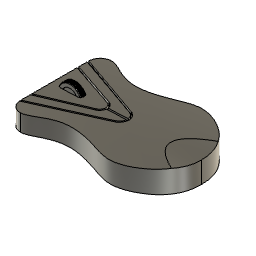
A4_AI22BTECH11005_4 (Autodesk Fusion 360 design; units mm, degrees)
Autodesk Fusion 360 part; units mm, degrees
sketch "Sketch1" plane through (0, 0, 0) normal (0, 0, 1) x (1, 0, 0)
  line L0 (0, 30) -> (0, -30)
  arc A0 (0, -30) -> (10, -40) centre (10, -30) ccw
  arc A1 (10, 40) -> (0, 30) centre (10, 30) ccw
  spline S0 degree 5 poles (10, 40) (10.9946, 40) (13.0682, 39.7459) (16.4315, 38.6027) (21.4876, 35.8702) (29.0437, 32.0592) (38.0149, 29.581) (48.2736, 29.5355) (59.1098, 31.6881) (69.5734, 35.0916) (78.8703, 38.4218) (86.7641, 40.4007) (93.9362, 40.1363) (102.6229, 37.6436) (112.4243, 32.71) (121.8387, 25.096) (127.3679, 16.6467) (129.5519, 8.8878) (130.0159, 3.0701) (130, 0) knots 0 0 0 0 0 0 0.066667 0.133333 0.2 0.266667 0.333333 0.4 0.466667 0.533333 0.6 0.666667 0.733333 0.8 0.866667 0.933333 1 1 1 1 1 1
  line L1 (2.9289, 40) -> (17.0711, 40)
  line L2 (27.8536, 31.0429) -> (52.1464, 28.9571)
  line L3 (82.1526, 40.1526) -> (97.8474, 39.8474)
  line L4 (130, 0) -> (0, 0)
  spline S1 degree 5 poles (10, -40) (10.9946, -40) (13.0682, -39.7459) (16.4315, -38.6027) (21.4876, -35.8702) (29.0437, -32.0592) (38.0149, -29.581) (48.2736, -29.5355) (59.1098, -31.6881) (69.5734, -35.0916) (78.8703, -38.4218) (86.7641, -40.4007) (93.9362, -40.1363) (102.6229, -37.6436) (112.4243, -32.71) (121.8387, -25.096) (127.3679, -16.6467) (129.5519, -8.8878) (130.0159, -3.0701) (130, 0) knots 0 0 0 0 0 0 0.066667 0.133333 0.2 0.266667 0.333333 0.4 0.466667 0.533333 0.6 0.666667 0.733333 0.8 0.866667 0.933333 1 1 1 1 1 1
  line L5 (130.0753, 14.5031) -> (129.9247, -14.5031)
  line L6 (2.9289, -40) -> (17.0711, -40)
  line L7 (27.8536, -31.0429) -> (52.1464, -28.9571)
  line L8 (82.1526, -40.1526) -> (97.8474, -39.8474)
  line L9 (130.0753, -14.5031) -> (129.9247, 14.5031)
  arc A2 (0, -30) -> (10, -40) centre (10, -30) ccw
  line L10 (0, -30) -> (0, 30)
  point P0 (130, 0)
  point P1 (40, 30)
  point P2 (90, 40)
  point P3 (40, -30)
  point P4 (90, -40)
  dimension "d1" = 10
  constraint vertical L0
  constraint tangent L0 A0
  constraint tangent L0 A1
  constraint equal A0 A1
  constraint coincident P0 S0.end
  constraint midpoint A1.start L1
  constraint tangent A1 L1
  constraint midpoint P1 L2
  constraint midpoint P2 L3
  constraint coincident L4.end origin
  constraint perpendicular L0 L4
  constraint midpoint P0 L5
  constraint symmetric L0.end L4 L0.start
  constraint symmetric L0.start L4 L0.end
  constraint symmetric A1.start L4 A0.end
  constraint symmetric A1 L4 A2
  constraint symmetric P1 L4 P3
  constraint symmetric P2 L4 P4
  constraint symmetric L1.start L4 L6.start
  constraint symmetric L1.end L4 L6.end
  constraint symmetric L2.start L4 L7.start
  constraint symmetric L2.end L4 L7.end
  constraint symmetric L3.start L4 L8.start
  constraint symmetric L3.end L4 L8.end
  constraint symmetric L4 L5.start L9.start
  constraint symmetric L4 L5.end L9.end
  measures "d1" radius of A0
extrude "Extrude1" add sketch "Sketch1" against normal blind 20
sketch "Sketch2" plane through (0, 0, 0) normal (0, 1, 0) x (1, 0, 0)
  line L0 (0, 0) -> (130.3347, 0)
  line L1 (130.3347, 0) -> (130.3347, 5.593)
  line L2 (130.3347, 5.593) -> (0, 5.593)
  line L3 (0, 5.593) -> (0, 0)
  line L4 (0, 5.593) -> (0, 0)
  line L5 (130.3347, 0) -> (130.3347, 5.593)
  line L6 (130.3347, 0) -> (65.1673, 0)
  line L7 (0, 5.593) -> (130.3347, 0)
  constraint coincident L0.start L3.end
  constraint horizontal L0
  constraint perpendicular L0 L1
  constraint perpendicular L1 L2
  constraint perpendicular L0 L3
  constraint midpoint L0 L6.end
extrude "Extrude2" cut sketch "Sketch2" along normal mid plane 100 contours L0 L3 L4 L6 L7
sketch "Sketch3" plane through (0, 0, 0) normal (0, 0, 1) x (1, 0, 0)
  line L0 (-1.0692, 29.9861, -8.2811) -> (-1.1456, -30.0143, -8.2905)
  line L1 (-1.0692, 29.9861, -8.2811) -> (61.0097, 7.0411, -0.6588)
  line L2 (61.0097, -7.0411, -0.6588) -> (-1.1456, -30.0143, -8.2905)
  arc A0 through (61.0097, -7.0411, -0.6588) (65.8899, 0, -0.0596) (61.0097, 7.0411, -0.6588)
  line L3 (0, -20) -> (0, 20)
  line L4 (0, -20) -> (42.0778, -4.699)
  line L5 (42.0778, 4.699) -> (0, 20)
  arc A1 (42.0778, -4.699) -> (42.0778, 4.699) centre (40.3691, 0) ccw
  line L6 (-1.3, -21.856) -> (-1.3, 21.856)
  line L7 (42.5221, 5.9207) -> (-1.3, 21.856)
  arc A2 (42.5221, -5.9207) -> (42.5221, 5.9207) centre (40.3691, 0) ccw
  line L8 (-1.3, -21.856) -> (42.5221, -5.9207)
  line L9 (46.6691, 0, 0) -> (65.8899, 0, -0.0596)
  line L10 (65.8024, 0) -> (65.8024, -0.75)
  line L11 (65.8024, -0.75) -> (45.9997, -0.75)
  line L12 (65.8024, 0.75) -> (65.8024, 0)
  line L13 (45.9997, 0.75) -> (45.9997, -0.75)
  line L14 (45.9997, 0.75) -> (65.8024, 0.75)
  line L15 (8.5721, 2.853) -> (23.7087, 2.853)
  line L16 (26.2087, 0.353) -> (26.2087, -0.647)
  line L17 (23.7087, -3.147) -> (8.5721, -3.147)
  line L18 (6.0721, 0.353) -> (6.0721, -0.647)
  arc A3 (8.5721, 2.853) -> (6.0721, 0.353) centre (8.5721, 0.353) ccw
  arc A4 (26.2087, 0.353) -> (23.7087, 2.853) centre (23.7087, 0.353) ccw
  arc A5 (23.7087, -3.147) -> (26.2087, -0.647) centre (23.7087, -0.647) ccw
  arc A6 (6.0721, -0.647) -> (8.5721, -3.147) centre (8.5721, -0.647) ccw
  line L19 (6.0721, -0.0328) -> (26.2087, -0.0328)
  line L20 (16.1404, -0.0328) -> (16.1404, 2.4672)
  line L21 (16.1404, -0.0328) -> (16.1404, -2.5328)
  line L22 (65.8024, 0, 0) -> (-0.9655, -29.9477, -8.2684)
  line L23 (85, 0, 0) -> (-1.1453, -29.7384, -8.2905)
  point P0 (66.9185, 0)
  point P1 (45.0032, -0.0207)
  point P2 (26.2087, 2.853)
  point P3 (26.2087, -3.147)
  point P4 (108.295, 0)
  dimension "d6" = 7.5
  dimension "d10" = 40
  dimension "d11" = 5
  dimension "d12" = 1.3
  dimension "d14" = 0.75
  dimension "d18" = 6
  dimension "d22" = 2.5
  dimension "d23" = 2.5
  dimension "d24" = 2.5
  constraint vertical L3
  constraint tangent L4 A1
  constraint tangent L5 A1
  constraint perpendicular L11 L13
  constraint horizontal L15
  constraint perpendicular L15 L16
  constraint perpendicular L16 L17
  constraint perpendicular L17 L18
  constraint tangent L15 A3
  constraint tangent L18 A3
  constraint coincident P2 L15
  constraint coincident P2 L16
  constraint tangent L15 A4
  constraint tangent L16 A4
  constraint equal A3 A4
  constraint coincident P3 L16
  constraint coincident P3 L17
  constraint tangent L16 A5
  constraint tangent L17 A5
  constraint equal A3 A5
  constraint tangent L17 A6
  constraint tangent L18 A6
  constraint equal A3 A6
  constraint coincident L18 L19.start
  constraint coincident L16 L19.end
  constraint perpendicular L16 L19
  constraint midpoint L19 L20.start
  constraint perpendicular L15 L20
  constraint perpendicular L19 L21
  measures "d10" distance of L3.start L3.end
  measures "d11" radius of A1
  measures "d14" distance of L10.start L10.end
  measures "d18" distance of P2 P3
  measures "d22" radius of A3
  measures "d23" distance of L20.start L20.end
  measures "d24" distance of L20.start L21.end
extrude "Extrude4" cut sketch "Sketch3" along normal mid plane 14 contours L6 L7 A2 L8 L11 L13 L14 | A2 L11 L13 L14 | A2 L10 L11 L12 L14
extrude "Extrude5" cut sketch "Sketch3" against normal blind 12 contours L15 L16 L18 A3 A4 L19 | L16 L17 L18 A5 A6 L19
ref_plane "WorkPlane1" through (16.1404, 1.2172, 0) normal (1, 0, 0) x (0, 1, 0)
sketch "Sketch5" plane through (16.1404, 1.2172, 0) normal (1, 0, 0) x (0, 1, 0)
  line L0 (1.25, 0) -> (1.25, -1.9482)
  line L1 (1.25, 0) -> (1.25, 1)
  line L2 (-3.75, 0) -> (-3.75, 1)
  line L3 (-3.75, 0) -> (-3.75, -1.9758)
  line L4 (-2.75, -9) -> (0.25, -9)
  arc A0 (1.25, 1) -> (0.75, 1.5) centre (0.75, 1) ccw
  arc A1 (-3.25, 1.5) -> (-3.75, 1) centre (-3.25, 1) ccw
  line L5 (1.25, -1.9482) -> (0.25, -1.9482)
  line L6 (0.25, -1.9482) -> (0.25, -9)
  line L7 (-3.75, -1.9758) -> (-2.75, -1.9758)
  line L8 (-2.75, -1.9758) -> (-2.75, -9)
  line L9 (-1.93, -1.5) -> (-2.0076, -1.5)
  line L10 (-2.9954, -1.4863) -> (-2.9954, 1.5)
  line L11 (-2.4997, -1.4863) -> (-2.4997, 1.5)
  line L12 (0.5056, 1.5) -> (0.5056, -1.4863)
  line L13 (0.017, 1.5) -> (0.017, -1.4863)
  line L14 (-0.5066, 1.5) -> (-0.5066, -1.4863)
  line L15 (-1.0186, 1.5) -> (-1.0186, -1.4863)
  line L16 (-1.5189, 1.5) -> (-1.5189, -1.4863)
  line L17 (-2.0076, 1.5) -> (-2.0076, -1.5)
  line L18 (0.75, 1.5) -> (0.5056, 1.5)
  line L19 (0.017, 1.5) -> (-0.5066, 1.5)
  line L20 (-1.0186, 1.5) -> (-1.5189, 1.5)
  line L21 (-2.0076, 1.5) -> (-2.4997, 1.5)
  line L22 (-2.9954, 1.5) -> (-3.25, 1.5)
  line L23 (0.017, -1.4863) -> (0.5056, -1.4863)
  line L24 (-1.0186, -1.4863) -> (-0.5066, -1.4863)
  line L25 (-2.9954, -1.4863) -> (-2.4997, -1.4863)
  line L26 (-2.0076, -1.4863) -> (-1.5189, -1.4863)
  point P0 (-3.75, 0)
  point P1 (1.25, 0)
  point P2 (1.25, 1.5)
  point P3 (-3.75, 1.5)
  dimension "d47" = 1.5
  dimension "d48" = 0.5
  dimension "d49" = 0.5
  dimension "d65" = 1
  dimension "d66" = 1
  constraint coincident P1 L0.start
  constraint vertical L0
  constraint parallel L0 L1
  constraint coincident P0 L2.start
  constraint vertical L2
  constraint parallel L2 L3
  constraint perpendicular L0 L4
  constraint coincident P2 L1
  constraint tangent L1 A0
  constraint coincident P3 L2
  constraint tangent L2 A1
  constraint perpendicular L0 L5
  constraint perpendicular L4 L6
  constraint perpendicular L3 L7
  constraint perpendicular L4 L8
  constraint tangent A1 L18
  constraint perpendicular L0 L25
  constraint coincident L10.end L18
  constraint perpendicular L10 L18
  constraint coincident L11.end L18
  constraint perpendicular L11 L18
  constraint coincident L12.end L25
  constraint perpendicular L12 L25
  constraint coincident L13.start L18
  constraint coincident L13.end L25
  constraint perpendicular L13 L25
  constraint coincident L14.start L18
  constraint perpendicular L14 L25
  constraint coincident L15.start L18
  constraint coincident L15.end L25
  constraint perpendicular L15 L25
  constraint coincident L16.start L18
  constraint perpendicular L16 L25
  constraint coincident L17.start L18
  constraint perpendicular L9 L17
  constraint collinear L18 L19
  constraint collinear L19 L20
  constraint collinear L20 L21
  constraint collinear L21 L22
  constraint collinear L23 L25
  constraint collinear L24 L25
  constraint coincident L17 L26.start
  constraint collinear L25 L26
  measures "d47" distance of P0 P3
  measures "d48" radius of A0
  measures "d49" radius of A1
  measures "d65" distance of L0.end L5.end
  measures "d66" distance of L3.end L7.end
revolve "Revolve2" add sketch "Sketch5" angle 360 about axis through (16.1404, -1.5328, -9) along (0, 1, 0)
ref_plane "WorkPlane4" through (100, 0, 0) normal (1, 0, 0) x (0, 1, 0)
sketch "Sketch8" plane through (100, 0, 0) normal (1, 0, 0) x (0, 1, 0)
  line L0 (-70, 10) -> (75, 10)
  line L1 (-70, 10) -> (-75, 10)
  spline S0 degree 5 poles (-75, 10) (-72.0002, 9.1521) (-66.0004, 7.5303) (-57.0008, 5.3198) (-45.0013, 2.824) (-30.0017, 0.5082) (-15.002, -0.932) (-0.0021, -1.425) (14.998, -0.9319) (29.9983, 0.5083) (44.9987, 2.8241) (56.9992, 5.3198) (65.9996, 7.5303) (71.9998, 9.1521) (75, 10) knots 0 0 0 0 0 0 0.1 0.2 0.3 0.4 0.5 0.6 0.7 0.8 0.9 1 1 1 1 1 1
  point P0 (-0.0039, -1.1792)
  dimension "d74" = 5
  constraint horizontal L0
  constraint parallel L0 L1
  measures "d74" distance of L0.start L1.end
extrude "Extrude7" cut sketch "Sketch8" along normal blind 50
ref_plane "WorkPlane5" through (0, 12.125, 0) normal (-0.034899, 0, 0.999391) x (0, 1, 0)
sketch "Sketch9" plane through (0, 12.125, 0) normal (-0.034899, 0, 0.999391) x (0, 1, 0)
  line L0 (20, 5) -> (-4.628, -60.418)
  line L1 (-19.5726, -60.4947) -> (-45, 5)
  line L2 (-45, 5) -> (20, 5)
  arc A0 (-19.5726, -60.4947) -> (-4.628, -60.418) centre (-12.115, -57.5994) ccw
  line L3 (18.1215, 3.7) -> (-5.8446, -59.96)
  arc A1 (-18.3608, -60.0242) -> (-5.8446, -59.96) centre (-12.115, -57.5994) ccw
  line L4 (-18.3608, -60.0242) -> (-43.1008, 3.7)
  line L5 (-43.1008, 3.7) -> (18.1215, 3.7)
  dimension "d78" = 8
  dimension "d79" = 1.3
  constraint horizontal L2
  constraint tangent L0 A0
  constraint tangent L1 A0
  measures "d78" radius of A0
extrude "Extrude8" cut sketch "Sketch9" against normal blind 7
